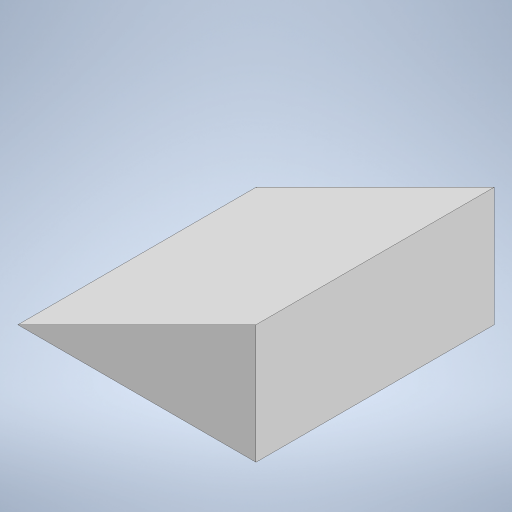
# Autodesk Inventor part: wedge
Saved by Autodesk Inventor 2023 (Build 270158000, 158)
## iProperties
Created: 2023-11-29
Part Number: wedge
Material: Generic
Document SubType Name: Modeling
Designer: Gage
Density: 1 g/cm^3
Appearance: Default
Author: Gage
Autodesk Inventor part; units mm, degrees
ref_plane "YZ Plane" through (0, 0, 0) normal (1, 0, 0) x (0, 1, 0)
ref_plane "XZ Plane" through (0, 0, 0) normal (0, 1, 0) x (-1, 0, 0)
ref_plane "XY Plane" through (0, 0, 0) normal (0, 0, 1) x (1, 0, 0)
sketch "Sketch1" plane through (0, 0, 0) normal (0, 0, 1) x (1, 0, 0)
  line L0 (31.75, 7.9375) -> (31.75, -17.4625)
  line L1 (31.75, -17.4625) -> (-19.05, -17.4625)
  line L2 (-19.05, -17.4625) -> (31.75, 7.9375)
  point P0 (0, 0)
  constraints: 6 end point
extrude "Extrusion1" add sketch "Sketch1" along normal blind 50.8
body "Solid1"
